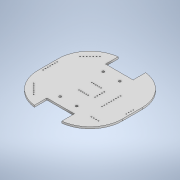
# Autodesk Inventor part: board_base
Saved by Autodesk Inventor 2020.3 (Build 243373000, 373)
## iProperties
Created: 2021-03-17
Part Number: board_base
Material: Ogólny
Document SubType Name: Modeling
Designer: patry
Density: 1 g/cm^3
Appearance: Domyślna
Author: patry
Autodesk Inventor part; units mm, degrees
ref_plane "YZ Plane" through (0, 0, 0) normal (1, 0, 0) x (0, 1, 0)
ref_plane "XZ Plane" through (0, 0, 0) normal (0, 1, 0) x (-1, 0, 0)
ref_plane "XY Plane" through (0, 0, 0) normal (0, 0, 1) x (1, 0, 0)
sketch "Szkic1" plane through (0, 0, 0) normal (0, 1, 0) x (-1, 0, 0)
  line L0 (11, 46) -> (-11, 46)
  line L1 (-46, 11) -> (-46, -11)
  line L2 (-11, -46) -> (11, -46)
  line L3 (46, -11) -> (46, 11)
  line L4 (46, 46) -> (-46, -46) construction
  line L5 (-46, 46) -> (46, -46) construction
  arc A0 (46, 44) -> (44, 46) centre (44, 44) ccw
  arc A1 (46, 11) -> (11, 46) centre (11, 11) ccw
  arc A2 (11, -46) -> (46, -11) centre (11, -11) ccw
  arc A3 (-46, -11) -> (-11, -46) centre (-11, -11) ccw
  arc A4 (-11, 46) -> (-46, 11) centre (-11, 11) ccw
  point P0 (0, 0)
  dimension "d0" = 92
  dimension "d1" = 92
  dimension "d3" = 35
  constraints: 12 end point, 10 point on circle, 10 point on line, 10 tangent, 5 centre point, 3 equal radius, 2 midpoint, 2 parallel, 1 horizontal, 1 perpendicular
  measures "d0" distance of L5.end L4.end
  measures "d1" distance of L4.end L5.start
  measures "d3" radius of A1
extrude "Wyciągnięcie proste1" add sketch "Szkic1" along normal blind 2
sketch "Szkic2" plane through (0, 2, 0) normal (0, 1, 0) x (1, 0, 0)
  line L0 (0, -49.4552) -> (0, 63.4462) construction
  line L1 (-44.5279, 0) -> (46.4745, 0) construction
  line L2 (15, 32) -> (-15, 32)
  line L3 (-15, 32) -> (-15, 46)
  line L4 (-15, 46) -> (15, 46)
  line L5 (15, 46) -> (15, 32)
  line L6 (15, 32) -> (-15, 46) construction
  line L7 (-15, 32) -> (15, 46) construction
  arc A0 (11, -46) -> (46, -11) centre (11, -11) ccw projected
  line L8 (46, -11) -> (46, 11) projected
  arc A1 (46, 11) -> (11, 46) centre (11, 11) ccw projected
  line L9 (11, 46) -> (-11, 46) projected
  arc A2 (-11, 46) -> (-46, 11) centre (-11, 11) ccw projected
  line L10 (-46, 11) -> (-46, -11) projected
  arc A3 (-46, -11) -> (-11, -46) centre (-11, -11) ccw projected
  line L11 (-11, -46) -> (11, -46) projected
  line L12 (11, 46) -> (-11, 46) projected
  line L13 (15, -46) -> (-15, -46)
  line L14 (-15, -46) -> (-15, -32)
  line L15 (-15, -32) -> (15, -32)
  line L16 (15, -32) -> (15, -46)
  line L17 (15, -46) -> (-15, -32) construction
  line L18 (-15, -46) -> (15, -32) construction
  line L19 (-11, -46) -> (11, -46) projected
  point P0 (0, 0)
  point P1 (0, 39)
  point P2 (0, -39)
  point P3 (0, -39)
  point P4 (0, 39)
  point P5 (-16, -46)
  point P6 (16, -46)
  dimension "d6" = 30
  dimension "d7" = 14
  dimension "d8" = 30
  dimension "d9" = 14
  constraints: 28 end point, 6 midpoint, 4 horizontal, 4 parallel, 2 collinear, 2 perpendicular, 2 vertical, 2 vertical alignment, 1 point on line
  measures "d6" distance of L3.end L4.end
  measures "d7" distance of L2.end L3.end
  measures "d8" distance of L15.start L15.end
  measures "d9" distance of L18.start L15.start
extrude "Wyciągnięcie proste2" cut sketch "Szkic2" against normal blind 10 contours L2 L3 A2 L4 A1 L5 | A1 L4 L5 | L3 L4 A2 | L16 L13 A0 | A0 L11 A3 L14 L15 L16 | A3 L13 L14
sketch "Szkic3" plane through (0, 2, 0) normal (0, 1, 0) x (1, 0, 0)
  line L0 (-15, -32) -> (15, -32) projected
  line L1 (-50.9262, 0) -> (55.7428, 0) construction
  point P0 (0, 0)
  point P1 (-9, -23.5)
  point P2 (9, -23.5)
  point P3 (-9, 23.5)
  point P4 (9, 23.5)
  dimension "d12" = 8.5
  dimension "d13" = 18
  dimension "d14" = 9
  constraints: 2 end point, 2 symmetric about line, 1 horizontal, 1 horizontal alignment
  measures "d12" distance from line of L0 point (-9, -23.5)
  measures "d13" distance of point (9, -23.5) point (-9, -23.5)
  measures "d14" horizontal distance of point (0, 0) point (-9, -23.5)
hole "Otwór1" at (-9, 2, 23.5) at (9, 2, 23.5) at (-9, 2, -23.5) at (9, 2, -23.5) direction (0, -1, 0) diameter 2.4 end through all clearance for "Śruba ze łbem płaskim obrobiona" size "M2" standard "ANSI Profil metryczny M"
sketch "Szkic4" plane through (0, 2, 0) normal (0, 1, 0) x (1, 0, 0)
  line L0 (-46, 11) -> (-46, -11) projected
  circle A0 centre (0, 0) radius 43.5 construction
  line L1 (-36.1473, 25.371) -> (-25.371, 36.1473) construction
  line L2 (-25.371, 36.1473) -> (-30.7591, 30.7591) construction
  line L3 (-43.5, 7.62) -> (-43.5, -7.62) construction
  line L4 (-50.7703, 0) -> (45.9031, 0) construction
  line L5 (-36.1473, -25.371) -> (-25.371, -36.1473) construction
  line L6 (-25.371, -36.1473) -> (-30.7591, -30.7591) construction
  point P0 (-43.5, 0)
  point P1 (-43.5, 2.54)
  point P2 (-43.5, -2.54)
  point P3 (-43.5, 5.08)
  point P4 (-43.5, -5.08)
  point P5 (-34.3512, 27.167)
  point P6 (-32.5552, 28.9631)
  point P7 (-27.167, 34.3512)
  point P8 (-28.9631, 32.5552)
  point P9 (-34.3512, -27.167)
  point P10 (-32.5552, -28.9631)
  point P11 (-27.167, -34.3512)
  point P12 (-28.9631, -32.5552)
  dimension "d22" = 2.54
  dimension "d23" = 2.54
  dimension "d24" = 2.54
  dimension "d25" = 2.54
  dimension "d26" = 2.54
  dimension "d27" = 2.54
  dimension "d28" = 2.5
  dimension "d36" = 15.24
  dimension "d37" = 7.62
  dimension "d38" = 135
  dimension "d39" = 5.3882
  dimension "d40" = 1.796
  dimension "d41" = 1.796
  dimension "d42" = 1.796
  dimension "d43" = 1.796
  constraints: 12 end point, 10 symmetric about line, 8 point on line, 7 coincident, 6 vertical alignment, 2 midpoint, 2 point on circle, 1 centre point, 1 horizontal, 1 horizontal alignment, 1 tangent, 1 vertical
  measures "d22" distance of A0.start point (-43.5, -2.54)
  measures "d23" distance of point (-43.5, 2.54) A0.start
  measures "d24" distance of point (-43.5, 5.08) point (-43.5, 2.54)
  measures "d25" distance of L3.start point (-43.5, 5.08)
  measures "d26" distance of point (-43.5, -5.08) point (-43.5, -2.54)
  measures "d27" distance of L3.end point (-43.5, -5.08)
  measures "d28" distance from line of L0 point (-43.5, -5.08)
  measures "d36" distance of L1.start L1.end
  measures "d37" distance of L2.start L2.end
  measures "d38" angle of L3 L1
  measures "d39" horizontal distance of L2.start L2.end
  measures "d40" horizontal distance of L2.start point (-27.167, 34.351)
  measures "d41" horizontal distance of A0.end point (-28.963, 32.555)
  measures "d42" horizontal distance of A0.end point (-32.555, 28.963)
  measures "d43" horizontal distance of point (-34.351, 27.167) point (-36.147, 25.371)
hole "Otwór2" at (-43.5, 2, 0) at (-43.5, 2, -2.54) at (-43.5, 2, 2.54) at (-43.5, 2, -5.08) at (-43.5, 2, 5.08) at (-43.5, 2, 7.62) at (-43.5, 2, -7.62) at (-36.1473, 2, 25.371) at (-30.7591, 2, 30.7591) at (-34.3512, 2, 27.167) at (-32.5552, 2, 28.9631) at (-27.167, 2, 34.3512) at (-28.9631, 2, 32.5552) at (-25.371, 2, 36.1473) at (-28.9631, 2, -32.5552) at (-27.167, 2, -34.3512) at (-32.5552, 2, -28.9631) at (-34.3512, 2, -27.167) at (-30.7591, 2, -30.7591) at (-25.371, 2, -36.1473) at (-36.1473, 2, -25.371) direction (0, -1, 0) diameter 1 end through all
sketch "Szkic5" plane through (0, 2, 0) normal (0, 1, 0) x (1, 0, 0)
  circle A0 centre (-25.371, 36.1473) radius 0.5 projected
  circle A1 centre (-34.3512, 27.167) radius 0.5 projected
  circle A2 centre (-27.167, 34.3512) radius 0.5 projected
  circle A3 centre (-25.371, -36.1473) radius 0.5 projected
  circle A4 centre (-27.167, -34.3512) radius 0.5 projected
  circle A5 centre (-34.3512, -27.167) radius 0.5 projected
  circle A6 centre (-36.1473, -25.371) radius 0.5 projected
  circle A7 centre (-43.5, -7.62) radius 0.5 projected
  circle A8 centre (-43.5, 5.08) radius 0.5 projected
  circle A9 centre (-43.5, 2.54) radius 0.5 projected
  circle A10 centre (-43.5, 0) radius 0.5 projected
  circle A11 centre (-43.5, -2.54) radius 0.5 projected
  circle A12 centre (-43.5, -5.08) radius 0.5 projected
  circle A13 centre (-43.5, 7.62) radius 0.5 projected
  circle A14 centre (-30.7591, -30.7591) radius 0.5 projected
  circle A15 centre (-32.5552, -28.9631) radius 0.5 projected
  circle A16 centre (-28.9631, -32.5552) radius 0.5 projected
  circle A17 centre (-28.9631, 32.5552) radius 0.5 projected
  circle A18 centre (-32.5552, 28.9631) radius 0.5 projected
  circle A19 centre (-30.7591, 30.7591) radius 0.5 projected
  circle A20 centre (-36.1473, 25.371) radius 0.5 projected
  circle A21 centre (-9, 23.5) radius 1.2 projected
  circle A22 centre (-9, -23.5) radius 1.2 projected
  circle A23 centre (9, -23.5) radius 1.2 projected
  circle A24 centre (9, 23.5) radius 1.2 projected
  line L0 (-15, 32) -> (-15, 45.7707) projected
  arc A25 (-15, 45.7707) -> (-46, 11) centre (-11, 11) ccw projected
  line L1 (-46, 11) -> (-46, -11) projected
  arc A26 (-46, -11) -> (-15, -45.7707) centre (-11, -11) ccw projected
  line L2 (-15, -45.7707) -> (-15, -32) projected
  line L3 (-15, -32) -> (15, -32) projected
  line L4 (15, -32) -> (15, -45.7707) projected
  arc A27 (15, -45.7707) -> (46, -11) centre (11, -11) ccw projected
  line L5 (46, -11) -> (46, 11) projected
  arc A28 (46, 11) -> (15, 45.7707) centre (11, 11) ccw projected
  line L6 (15, 45.7707) -> (15, 32) projected
  line L7 (15, 32) -> (-15, 32) projected
  line L8 (7.5, -32) -> (-7.5, -32)
  line L9 (-7.5, -32) -> (-7.5, -18.75)
  line L10 (-7.5, -18.75) -> (7.5, -18.75)
  line L11 (7.5, -18.75) -> (7.5, -32)
  line L12 (7.5, -32) -> (-7.5, -18.75) construction
  line L13 (-7.5, -32) -> (7.5, -18.75) construction
  line L14 (-15, -32) -> (15, -32) projected
  circle A29 centre (-9, -23.5) radius 4.25
  line L15 (-9, -19.25) -> (-7.5, -19.25)
  line L16 (-9, -27.75) -> (-7.5, -27.75)
  circle A30 centre (9, -23.5) radius 1.2 projected
  circle A31 centre (9, -23.5) radius 4.25
  line L17 (9, -19.25) -> (7.5, -19.25)
  line L18 (9, -27.75) -> (7.5, -27.75)
  line L19 (6, -18.75) -> (-6, -18.75)
  line L20 (-6, -18.75) -> (-6, -10.25)
  line L21 (-6, -10.25) -> (6, -10.25)
  line L22 (6, -10.25) -> (6, -18.75)
  line L23 (6, -18.75) -> (-6, -10.25) construction
  line L24 (-6, -18.75) -> (6, -10.25) construction
  line L25 (0.5, -10.25) -> (-0.5, -10.25)
  line L26 (-0.5, -10.25) -> (-0.5, -5.25)
  line L27 (-0.5, -5.25) -> (0.5, -5.25)
  line L28 (0.5, -5.25) -> (0.5, -10.25)
  line L29 (0.5, -10.25) -> (-0.5, -5.25) construction
  line L30 (-0.5, -10.25) -> (0.5, -5.25) construction
  line L31 (-48.5218, 0) -> (66.2136, 0) construction
  circle A32 centre (-9, 23.5) radius 1.2
  circle A33 centre (9, 23.5) radius 1.2
  line L32 (7.5, 32) -> (-7.5, 32)
  line L33 (-7.5, 32) -> (-7.5, 18.75)
  line L34 (-7.5, 18.75) -> (7.5, 18.75)
  line L35 (7.5, 18.75) -> (7.5, 32)
  line L36 (7.5, 32) -> (-7.5, 18.75) construction
  line L37 (-7.5, 32) -> (7.5, 18.75) construction
  line L38 (-9, 19.25) -> (-7.5, 19.25)
  line L39 (-9, 27.75) -> (-7.5, 27.75)
  circle A34 centre (9, 23.5) radius 1.2
  circle A35 centre (9, 23.5) radius 4.25
  line L40 (9, 19.25) -> (7.5, 19.25)
  line L41 (9, 27.75) -> (7.5, 27.75)
  line L42 (6, 18.75) -> (-6, 18.75)
  line L43 (-6, 18.75) -> (-6, 10.25)
  line L44 (-6, 10.25) -> (6, 10.25)
  line L45 (6, 10.25) -> (6, 18.75)
  line L46 (6, 18.75) -> (-6, 10.25) construction
  line L47 (-6, 18.75) -> (6, 10.25) construction
  line L48 (0.5, 10.25) -> (-0.5, 10.25)
  line L49 (-0.5, 10.25) -> (-0.5, 5.25)
  line L50 (-0.5, 5.25) -> (0.5, 5.25)
  line L51 (0.5, 5.25) -> (0.5, 10.25)
  line L52 (0.5, 10.25) -> (-0.5, 5.25) construction
  line L53 (-0.5, 10.25) -> (0.5, 5.25) construction
  circle A36 centre (-9, 23.5) radius 4.25
  point P0 (0, 0)
  point P1 (0, -25.375)
  point P2 (0, -25.375)
  point P3 (0, -14.5)
  point P4 (0, -14.5)
  point P5 (0, -25.375)
  point P6 (0, -7.75)
  point P7 (0, -7.75)
  point P8 (-1, -7)
  point P9 (-3, -7)
  point P10 (-5, -7)
  point P11 (1, -7)
  point P12 (3, -7)
  point P13 (5, -7)
  point P14 (0, 25.375)
  point P15 (0, 25.375)
  point P16 (0, 14.5)
  point P17 (0, 14.5)
  point P18 (0, 25.375)
  point P19 (0, 7.75)
  point P20 (0, 7.75)
  point P21 (-1, 7)
  point P22 (-3, 7)
  point P23 (-5, 7)
  point P24 (1, 7)
  point P25 (3, 7)
  point P26 (5, 7)
  dimension "d44" = 15
  dimension "d45" = 13.25
  dimension "d46" = 8.5
  dimension "d47" = 8.5
  dimension "d48" = 12
  dimension "d49" = 8.5
  dimension "d50" = 1
  dimension "d51" = 5
  dimension "d53" = 2
  dimension "d54" = 2
  dimension "d55" = 2
  dimension "d56" = 2
  dimension "d57" = 2
  dimension "d58" = 1
  dimension "d59" = 3.25
  constraints: 90 end point, 39 symmetric about line, 16 midpoint, 8 point on line, 7 centre point, 7 perpendicular, 6 parallel, 6 point on circle, 5 horizontal alignment, 4 coincident, 4 horizontal, 3 collinear, 3 vertical alignment, 5 other
  measures "d44" distance of L9.end L10.end
  measures "d45" distance of L8.end L9.end
  measures "d46" diameter of A29
  measures "d47" diameter of A31
  measures "d48" distance of L20.end L21.end
  measures "d49" distance of L19.end L20.end
  measures "d50" distance of L26.end L27.end
  measures "d51" distance of L25.end L26.end
  measures "d53" distance of point (1, -7) point (-1, -7)
  measures "d54" distance of point (-1, -7) point (-3, -7)
  measures "d55" distance of point (-3, -7) point (-5, -7)
  measures "d56" distance of point (1, -7) point (3, -7)
  measures "d57" distance of point (3, -7) point (5, -7)
  measures "d58" horizontal distance of point (-1, -7) point (0, -7.75)
  measures "d59" distance from line of L21 point (-1, -7)
hole "Otwór3" at (-1, 2, 7) at (-3, 2, 7) at (-5, 2, 7) at (1, 2, 7) at (3, 2, 7) at (5, 2, 7) at (5, 2, -7) at (3, 2, -7) at (1, 2, -7) at (-5, 2, -7) at (-3, 2, -7) at (-1, 2, -7) direction (0, -1, 0) diameter 1 end through all
sketch "Szkic6" plane through (0, 2, 0) normal (0, 1, 0) x (1, 0, 0)
  circle A0 centre (-3, 7) radius 0.5 projected
  circle A1 centre (1, 7) radius 0.5 projected
  circle A2 centre (5, 7) radius 0.5 projected
  circle A3 centre (3, -7) radius 0.5 projected
  circle A4 centre (-5, -7) radius 0.5 projected
  circle A5 centre (-1, -7) radius 0.5 projected
  circle A6 centre (-3, -7) radius 0.5 projected
  circle A7 centre (1, -7) radius 0.5 projected
  circle A8 centre (5, -7) radius 0.5 projected
  circle A9 centre (3, 7) radius 0.5 projected
  circle A10 centre (-5, 7) radius 0.5 projected
  circle A11 centre (-1, 7) radius 0.5 projected
  circle A12 centre (-25.371, 36.1473) radius 0.5 projected
  circle A13 centre (-34.3512, 27.167) radius 0.5 projected
  circle A14 centre (-27.167, 34.3512) radius 0.5 projected
  circle A15 centre (-25.371, -36.1473) radius 0.5 projected
  circle A16 centre (-27.167, -34.3512) radius 0.5 projected
  circle A17 centre (-34.3512, -27.167) radius 0.5 projected
  circle A18 centre (-36.1473, -25.371) radius 0.5 projected
  circle A19 centre (-43.5, -7.62) radius 0.5 projected
  circle A20 centre (-43.5, 5.08) radius 0.5 projected
  circle A21 centre (-43.5, 2.54) radius 0.5 projected
  circle A22 centre (-43.5, 0) radius 0.5 projected
  circle A23 centre (-43.5, -2.54) radius 0.5 projected
  circle A24 centre (-43.5, -5.08) radius 0.5 projected
  circle A25 centre (-43.5, 7.62) radius 0.5 projected
  circle A26 centre (-30.7591, -30.7591) radius 0.5 projected
  circle A27 centre (-32.5552, -28.9631) radius 0.5 projected
  circle A28 centre (-28.9631, -32.5552) radius 0.5 projected
  circle A29 centre (-28.9631, 32.5552) radius 0.5 projected
  circle A30 centre (-32.5552, 28.9631) radius 0.5 projected
  circle A31 centre (-30.7591, 30.7591) radius 0.5 projected
  circle A32 centre (-36.1473, 25.371) radius 0.5 projected
  circle A33 centre (-9, 23.5) radius 1.2 projected
  circle A34 centre (-9, -23.5) radius 1.2 projected
  circle A35 centre (9, -23.5) radius 1.2 projected
  circle A36 centre (9, 23.5) radius 1.2 projected
  line L0 (-15, 32) -> (-15, 45.7707) projected
  arc A37 (-15, 45.7707) -> (-46, 11) centre (-11, 11) ccw projected
  line L1 (-46, 11) -> (-46, -11) projected
  arc A38 (-46, -11) -> (-15, -45.7707) centre (-11, -11) ccw projected
  line L2 (-15, -45.7707) -> (-15, -32) projected
  line L3 (-15, -32) -> (15, -32) projected
  line L4 (15, -32) -> (15, -45.7707) projected
  arc A39 (15, -45.7707) -> (46, -11) centre (11, -11) ccw projected
  line L5 (46, -11) -> (46, 11) projected
  arc A40 (46, 11) -> (15, 45.7707) centre (11, 11) ccw projected
  line L6 (15, 45.7707) -> (15, 32) projected
  line L7 (15, 32) -> (-15, 32) projected
  line L8 (25.8, -12.7) -> (8, -12.7)
  line L9 (8, -12.7) -> (8, 12.7)
  line L10 (8, 12.7) -> (25.8, 12.7)
  line L11 (25.8, 12.7) -> (25.8, -12.7)
  line L12 (25.8, -12.7) -> (8, 12.7) construction
  line L13 (8, -12.7) -> (25.8, 12.7) construction
  line L14 (6, 10.25) -> (6, 18.75) projected
  line L15 (6, -10.25) -> (6, -18.75) projected
  point P0 (0, 0)
  point P1 (16.9, 0)
  point P2 (16.9, 0)
  point P3 (10.55, 0)
  point P4 (23.25, 0)
  point P5 (10.55, 2.54)
  point P6 (10.55, 5.08)
  point P7 (10.55, -2.54)
  point P8 (10.55, -5.08)
  point P9 (23.25, 0)
  point P10 (23.25, 2.54)
  point P11 (23.25, 5.08)
  point P12 (23.25, -2.54)
  point P13 (23.25, -5.08)
  point P14 (23.25, 7.62)
  point P15 (23.25, 10.16)
  point P16 (23.25, -7.62)
  point P17 (23.25, -10.16)
  dimension "d67" = 17.8
  dimension "d68" = 25.4
  dimension "d69" = 2
  dimension "d70" = 6.35
  dimension "d71" = 6.35
  dimension "d72" = 2.54
  dimension "d73" = 2.54
  dimension "d74" = 2.54
  dimension "d75" = 2.54
  dimension "d76" = 2.54
  dimension "d77" = 2.54
  dimension "d78" = 2.54
  dimension "d79" = 2.54
  dimension "d80" = 2.54
  dimension "d82" = 2.54
  dimension "d83" = 2.54
  dimension "d85" = 2.54
  constraints: 12 end point, 12 vertical alignment, 3 midpoint, 2 parallel, 1 coincident, 1 horizontal, 1 horizontal alignment, 1 perpendicular
  measures "d67" distance of L9.end L10.end
  measures "d68" distance of L8.end L9.end
  measures "d69" distance between parallel lines of L9 L14
  measures "d70" distance of point (16.9, 0) point (10.55, 0)
  measures "d71" distance of point (16.9, 0) point (23.25, 0)
  measures "d72" distance of point (10.55, 2.54) point (10.55, 0)
  measures "d73" distance of point (10.55, 2.54) point (10.55, 5.08)
  measures "d74" distance of point (10.55, 0) point (10.55, -2.54)
  measures "d75" distance of point (10.55, -2.54) point (10.55, -5.08)
  measures "d76" distance of point (23.25, 2.54) point (23.25, 0)
  measures "d77" distance of point (23.25, 2.54) point (23.25, 5.08)
  measures "d78" distance of point (23.25, 0) point (23.25, -2.54)
  measures "d79" distance of point (23.25, -2.54) point (23.25, -5.08)
  measures "d80" distance of point (23.25, 10.16) point (23.25, 7.62)
  measures "d82" distance of point (23.25, 5.08) point (23.25, 7.62)
  measures "d83" distance of point (23.25, -10.16) point (23.25, -7.62)
  measures "d85" distance of point (23.25, -5.08) point (23.25, -7.62)
hole "Otwór4" at (10.55, 2, 5.08) at (10.55, 2, 2.54) at (10.55, 2, -5.08) at (10.55, 2, -2.54) at (10.55, 2, 0) at (23.25, 2, 7.62) at (23.25, 2, 10.16) at (23.25, 2, -7.62) at (23.25, 2, -10.16) at (23.25, 2, 0) at (23.25, 2, -2.54) at (23.25, 2, -5.08) at (23.25, 2, 2.54) at (23.25, 2, 5.08) direction (0, -1, 0) diameter 1 end through all
sketch "Szkic7" plane through (0, 2, 0) normal (0, 1, 0) x (1, 0, 0)
  circle A0 centre (23.25, -2.54) radius 0.5 projected
  circle A1 centre (23.25, 2.54) radius 0.5 projected
  circle A2 centre (23.25, 10.16) radius 0.5 projected
  circle A3 centre (23.25, -10.16) radius 0.5 projected
  circle A4 centre (10.55, 0) radius 0.5 projected
  circle A5 centre (10.55, 5.08) radius 0.5 projected
  circle A6 centre (10.55, -5.08) radius 0.5 projected
  circle A7 centre (10.55, -2.54) radius 0.5 projected
  circle A8 centre (10.55, 2.54) radius 0.5 projected
  circle A9 centre (23.25, -7.62) radius 0.5 projected
  circle A10 centre (23.25, 7.62) radius 0.5 projected
  circle A11 centre (23.25, 0) radius 0.5 projected
  circle A12 centre (23.25, 5.08) radius 0.5 projected
  circle A13 centre (23.25, -5.08) radius 0.5 projected
  circle A14 centre (-3, 7) radius 0.5 projected
  circle A15 centre (1, 7) radius 0.5 projected
  circle A16 centre (5, 7) radius 0.5 projected
  circle A17 centre (3, -7) radius 0.5 projected
  circle A18 centre (-5, -7) radius 0.5 projected
  circle A19 centre (-1, -7) radius 0.5 projected
  circle A20 centre (-3, -7) radius 0.5 projected
  circle A21 centre (1, -7) radius 0.5 projected
  circle A22 centre (5, -7) radius 0.5 projected
  circle A23 centre (3, 7) radius 0.5 projected
  circle A24 centre (-5, 7) radius 0.5 projected
  circle A25 centre (-1, 7) radius 0.5 projected
  circle A26 centre (-25.371, 36.1473) radius 0.5 projected
  circle A27 centre (-34.3512, 27.167) radius 0.5 projected
  circle A28 centre (-27.167, 34.3512) radius 0.5 projected
  circle A29 centre (-25.371, -36.1473) radius 0.5 projected
  circle A30 centre (-27.167, -34.3512) radius 0.5 projected
  circle A31 centre (-34.3512, -27.167) radius 0.5 projected
  circle A32 centre (-36.1473, -25.371) radius 0.5 projected
  circle A33 centre (-43.5, -7.62) radius 0.5 projected
  circle A34 centre (-43.5, 5.08) radius 0.5 projected
  circle A35 centre (-43.5, 2.54) radius 0.5 projected
  circle A36 centre (-43.5, 0) radius 0.5 projected
  circle A37 centre (-43.5, -2.54) radius 0.5 projected
  circle A38 centre (-43.5, -5.08) radius 0.5 projected
  circle A39 centre (-43.5, 7.62) radius 0.5 projected
  circle A40 centre (-30.7591, -30.7591) radius 0.5 projected
  circle A41 centre (-32.5552, -28.9631) radius 0.5 projected
  circle A42 centre (-28.9631, -32.5552) radius 0.5 projected
  circle A43 centre (-28.9631, 32.5552) radius 0.5 projected
  circle A44 centre (-32.5552, 28.9631) radius 0.5 projected
  circle A45 centre (-30.7591, 30.7591) radius 0.5 projected
  circle A46 centre (-36.1473, 25.371) radius 0.5 projected
  circle A47 centre (-9, 23.5) radius 1.2 projected
  circle A48 centre (-9, -23.5) radius 1.2 projected
  circle A49 centre (9, -23.5) radius 1.2 projected
  circle A50 centre (9, 23.5) radius 1.2 projected
  line L0 (-15, 32) -> (-15, 45.7707) projected
  arc A51 (-15, 45.7707) -> (-46, 11) centre (-11, 11) ccw projected
  line L1 (-46, 11) -> (-46, -11) projected
  arc A52 (-46, -11) -> (-15, -45.7707) centre (-11, -11) ccw projected
  line L2 (-15, -45.7707) -> (-15, -32) projected
  line L3 (-15, -32) -> (15, -32) projected
  line L4 (15, -32) -> (15, -45.7707) projected
  arc A53 (15, -45.7707) -> (46, -11) centre (11, -11) ccw projected
  line L5 (46, -11) -> (46, 11) projected
  arc A54 (46, 11) -> (15, 45.7707) centre (11, 11) ccw projected
  line L6 (15, 45.7707) -> (15, 32) projected
  line L7 (15, 32) -> (-15, 32) projected
  line L8 (-48.5218, 0) -> (66.2136, 0) construction
  point P0 (0, 0)
  point P1 (43.5, -1.27)
  point P2 (43.5, 1.27)
  point P3 (43.5, 3.81)
  point P4 (43.5, -3.81)
  dimension "d93" = 2.5
  dimension "d94" = 2.54
  dimension "d95" = 1.27
  dimension "d96" = 2.54
  dimension "d97" = 2.54
  constraints: 3 vertical alignment
  measures "d93" distance from line of L5 point (43.5, -1.27)
  measures "d94" distance of point (43.5, 1.27) point (43.5, -1.27)
  measures "d95" distance from line of L8 point (43.5, 1.27)
  measures "d96" distance of point (43.5, 3.81) point (43.5, 1.27)
  measures "d97" distance of point (43.5, -3.81) point (43.5, -1.27)
hole "Otwór5" at (43.5, 2, 3.81) at (43.5, 2, -3.81) at (43.5, 2, -1.27) at (43.5, 2, 1.27) direction (0, -1, 0) diameter 1 end through all
sketch "Szkic8" plane through (0, 2, 0) normal (0, 1, 0) x (1, 0, 0)
  line L0 (27.0445, -22.5) -> (42.0445, -22.5) construction
  line L1 (42.0445, -22.5) -> (42.0445, 22.5) construction
  line L2 (42.0445, 22.5) -> (27.0445, 22.5) construction
  line L3 (27.0445, 22.5) -> (27.0445, -22.5) construction
  line L4 (27.0445, -22.5) -> (42.0445, 22.5) construction
  line L5 (42.0445, -22.5) -> (27.0445, 22.5) construction
  point P0 (0, 0)
  point P1 (34.5445, 0)
  point P2 (27.0445, -25.5)
  point P3 (29.5845, -25.5)
  point P4 (32.1245, -25.5)
  point P5 (34.6645, -25.5)
  dimension "d105" = 15
  dimension "d106" = 45
  dimension "d107" = 2.54
  dimension "d108" = 2.54
  dimension "d109" = 2.54
  dimension "d110" = 3
  dimension "d111" = 0
  constraints: 12 end point, 3 horizontal alignment, 2 midpoint, 2 parallel, 1 horizontal, 1 perpendicular
  measures "d105" distance of L2.end L1.end
  measures "d106" distance of L1.end L0.end
  measures "d107" distance of point (29.585, -25.5) point (27.045, -25.5)
  measures "d108" distance of point (32.125, -25.5) point (29.585, -25.5)
  measures "d109" distance of point (34.665, -25.5) point (32.125, -25.5)
  measures "d110" distance from line of L0 point (27.045, -25.5)
  measures "d111" distance from line of L3 point (27.045, -25.5)
hole "Otwór6" at (34.6645, 2, 25.5) at (32.1245, 2, 25.5) at (29.5845, 2, 25.5) at (27.0445, 2, 25.5) direction (0, -1, 0) diameter 1 end through all
sketch "Szkic9" plane through (0, 2, 0) normal (0, 1, 0) x (1, 0, 0)
  circle A0 centre (29.5845, -25.5) radius 0.5 projected
  circle A1 centre (34.6645, -25.5) radius 0.5 projected
  circle A2 centre (32.1245, -25.5) radius 0.5 projected
  circle A3 centre (27.0445, -25.5) radius 0.5 projected
  circle A4 centre (43.5, 1.27) radius 0.5 projected
  circle A5 centre (43.5, -3.81) radius 0.5 projected
  circle A6 centre (43.5, 3.81) radius 0.5 projected
  circle A7 centre (43.5, -1.27) radius 0.5 projected
  circle A8 centre (23.25, -2.54) radius 0.5 projected
  circle A9 centre (23.25, 2.54) radius 0.5 projected
  circle A10 centre (23.25, 10.16) radius 0.5 projected
  circle A11 centre (23.25, -10.16) radius 0.5 projected
  circle A12 centre (10.55, 0) radius 0.5 projected
  circle A13 centre (10.55, 5.08) radius 0.5 projected
  circle A14 centre (10.55, -5.08) radius 0.5 projected
  circle A15 centre (10.55, -2.54) radius 0.5 projected
  circle A16 centre (10.55, 2.54) radius 0.5 projected
  circle A17 centre (23.25, -7.62) radius 0.5 projected
  circle A18 centre (23.25, 7.62) radius 0.5 projected
  circle A19 centre (23.25, 0) radius 0.5 projected
  circle A20 centre (23.25, 5.08) radius 0.5 projected
  circle A21 centre (23.25, -5.08) radius 0.5 projected
  circle A22 centre (-3, 7) radius 0.5 projected
  circle A23 centre (1, 7) radius 0.5 projected
  circle A24 centre (5, 7) radius 0.5 projected
  circle A25 centre (3, -7) radius 0.5 projected
  circle A26 centre (-5, -7) radius 0.5 projected
  circle A27 centre (-1, -7) radius 0.5 projected
  circle A28 centre (-3, -7) radius 0.5 projected
  circle A29 centre (1, -7) radius 0.5 projected
  circle A30 centre (5, -7) radius 0.5 projected
  circle A31 centre (3, 7) radius 0.5 projected
  circle A32 centre (-5, 7) radius 0.5 projected
  circle A33 centre (-1, 7) radius 0.5 projected
  circle A34 centre (-25.371, 36.1473) radius 0.5 projected
  circle A35 centre (-34.3512, 27.167) radius 0.5 projected
  circle A36 centre (-27.167, 34.3512) radius 0.5 projected
  circle A37 centre (-25.371, -36.1473) radius 0.5 projected
  circle A38 centre (-27.167, -34.3512) radius 0.5 projected
  circle A39 centre (-34.3512, -27.167) radius 0.5 projected
  circle A40 centre (-36.1473, -25.371) radius 0.5 projected
  circle A41 centre (-43.5, -7.62) radius 0.5 projected
  circle A42 centre (-43.5, 5.08) radius 0.5 projected
  circle A43 centre (-43.5, 2.54) radius 0.5 projected
  circle A44 centre (-43.5, 0) radius 0.5 projected
  circle A45 centre (-43.5, -2.54) radius 0.5 projected
  circle A46 centre (-43.5, -5.08) radius 0.5 projected
  circle A47 centre (-43.5, 7.62) radius 0.5 projected
  circle A48 centre (-30.7591, -30.7591) radius 0.5 projected
  circle A49 centre (-32.5552, -28.9631) radius 0.5 projected
  circle A50 centre (-28.9631, -32.5552) radius 0.5 projected
  circle A51 centre (-28.9631, 32.5552) radius 0.5 projected
  circle A52 centre (-32.5552, 28.9631) radius 0.5 projected
  circle A53 centre (-30.7591, 30.7591) radius 0.5 projected
  circle A54 centre (-36.1473, 25.371) radius 0.5 projected
  circle A55 centre (-9, 23.5) radius 1.2 projected
  circle A56 centre (-9, -23.5) radius 1.2 projected
  circle A57 centre (9, -23.5) radius 1.2 projected
  circle A58 centre (9, 23.5) radius 1.2 projected
  line L0 (-15, 32) -> (-15, 45.7707) projected
  arc A59 (-15, 45.7707) -> (-46, 11) centre (-11, 11) ccw projected
  line L1 (-46, 11) -> (-46, -11) projected
  arc A60 (-46, -11) -> (-15, -45.7707) centre (-11, -11) ccw projected
  line L2 (-15, -45.7707) -> (-15, -32) projected
  line L3 (-15, -32) -> (15, -32) projected
  line L4 (15, -32) -> (15, -45.7707) projected
  arc A61 (15, -45.7707) -> (46, -11) centre (11, -11) ccw projected
  line L5 (46, -11) -> (46, 11) projected
  arc A62 (46, 11) -> (15, 45.7707) centre (11, 11) ccw projected
  line L6 (15, 45.7707) -> (15, 32) projected
  line L7 (15, 32) -> (-15, 32) projected
  circle A63 centre (-9, 23.5) radius 4.25 projected
  circle A64 centre (9, 23.5) radius 4.25 projected
  line L8 (7.5, 18.75) -> (7.5, 32) projected
  line L9 (-7.5, 32) -> (-7.5, 18.75) projected
  line L10 (6, 18.75) -> (-6, 18.75) projected
  line L11 (-6, 18.75) -> (-6, 10.25) projected
  line L12 (-6, 10.25) -> (6, 10.25) projected
  line L13 (6, 10.25) -> (6, 18.75) projected
  circle A65 centre (-9, -23.5) radius 4.25 projected
  circle A66 centre (9, -23.5) radius 4.25 projected
  line L14 (7.5, -18.75) -> (7.5, -32) projected
  line L15 (-7.5, -32) -> (-7.5, -18.75) projected
  line L16 (-6, -18.75) -> (-6, -10.25) projected
  line L17 (-7.5, -18.75) -> (7.5, -18.75) projected
  line L18 (6, -10.25) -> (6, -18.75) projected
  line L19 (-6, -10.25) -> (6, -10.25) projected
  line L20 (0.5, 5.25) -> (0.5, 10.25) projected
  line L21 (-0.5, 10.25) -> (-0.5, 5.25) projected
  line L22 (-0.5, 5.25) -> (0.5, 5.25) projected
  line L23 (-0.5, -5.25) -> (0.5, -5.25) projected
  line L24 (-0.5, -10.25) -> (-0.5, -5.25) projected
  line L25 (0.5, -5.25) -> (0.5, -10.25) projected
  line L26 (27.0445, 22.5) -> (27.0445, -22.5) construction
  line L27 (42.0445, 22.5) -> (27.0445, 22.5) construction
  line L28 (42.0445, -22.5) -> (42.0445, 22.5) construction
  line L29 (27.0445, -22.5) -> (42.0445, -22.5) construction
  line L30 (25.8, 12.7) -> (25.8, -12.7) projected
  line L31 (8, 12.7) -> (25.8, 12.7) projected
  line L32 (8, -12.7) -> (8, 12.7) projected
  line L33 (25.8, -12.7) -> (8, -12.7) projected
  point P0 (0, 0)
sketch "Szkic10" plane through (0, 2, 0) normal (0, 1, 0) x (1, 0, 0)
  circle A0 centre (29.5845, -25.5) radius 0.5 projected
  circle A1 centre (34.6645, -25.5) radius 0.5 projected
  circle A2 centre (32.1245, -25.5) radius 0.5 projected
  circle A3 centre (27.0445, -25.5) radius 0.5 projected
  circle A4 centre (43.5, 1.27) radius 0.5 projected
  circle A5 centre (43.5, -3.81) radius 0.5 projected
  circle A6 centre (43.5, 3.81) radius 0.5 projected
  circle A7 centre (43.5, -1.27) radius 0.5 projected
  circle A8 centre (23.25, -2.54) radius 0.5 projected
  circle A9 centre (23.25, 2.54) radius 0.5 projected
  circle A10 centre (23.25, 10.16) radius 0.5 projected
  circle A11 centre (23.25, -10.16) radius 0.5 projected
  circle A12 centre (10.55, 0) radius 0.5 projected
  circle A13 centre (10.55, 5.08) radius 0.5 projected
  circle A14 centre (10.55, -5.08) radius 0.5 projected
  circle A15 centre (10.55, -2.54) radius 0.5 projected
  circle A16 centre (10.55, 2.54) radius 0.5 projected
  circle A17 centre (23.25, -7.62) radius 0.5 projected
  circle A18 centre (23.25, 7.62) radius 0.5 projected
  circle A19 centre (23.25, 0) radius 0.5 projected
  circle A20 centre (23.25, 5.08) radius 0.5 projected
  circle A21 centre (23.25, -5.08) radius 0.5 projected
  circle A22 centre (-3, 7) radius 0.5 projected
  circle A23 centre (1, 7) radius 0.5 projected
  circle A24 centre (5, 7) radius 0.5 projected
  circle A25 centre (3, -7) radius 0.5 projected
  circle A26 centre (-5, -7) radius 0.5 projected
  circle A27 centre (-1, -7) radius 0.5 projected
  circle A28 centre (-3, -7) radius 0.5 projected
  circle A29 centre (1, -7) radius 0.5 projected
  circle A30 centre (5, -7) radius 0.5 projected
  circle A31 centre (3, 7) radius 0.5 projected
  circle A32 centre (-5, 7) radius 0.5 projected
  circle A33 centre (-1, 7) radius 0.5 projected
  circle A34 centre (-25.371, 36.1473) radius 0.5 projected
  circle A35 centre (-34.3512, 27.167) radius 0.5 projected
  circle A36 centre (-27.167, 34.3512) radius 0.5 projected
  circle A37 centre (-25.371, -36.1473) radius 0.5 projected
  circle A38 centre (-27.167, -34.3512) radius 0.5 projected
  circle A39 centre (-34.3512, -27.167) radius 0.5 projected
  circle A40 centre (-36.1473, -25.371) radius 0.5 projected
  circle A41 centre (-43.5, -7.62) radius 0.5 projected
  circle A42 centre (-43.5, 5.08) radius 0.5 projected
  circle A43 centre (-43.5, 2.54) radius 0.5 projected
  circle A44 centre (-43.5, 0) radius 0.5 projected
  circle A45 centre (-43.5, -2.54) radius 0.5 projected
  circle A46 centre (-43.5, -5.08) radius 0.5 projected
  circle A47 centre (-43.5, 7.62) radius 0.5 projected
  circle A48 centre (-30.7591, -30.7591) radius 0.5 projected
  circle A49 centre (-32.5552, -28.9631) radius 0.5 projected
  circle A50 centre (-28.9631, -32.5552) radius 0.5 projected
  circle A51 centre (-28.9631, 32.5552) radius 0.5 projected
  circle A52 centre (-32.5552, 28.9631) radius 0.5 projected
  circle A53 centre (-30.7591, 30.7591) radius 0.5 projected
  circle A54 centre (-36.1473, 25.371) radius 0.5 projected
  circle A55 centre (-9, 23.5) radius 1.2 projected
  circle A56 centre (-9, -23.5) radius 1.2 projected
  circle A57 centre (9, -23.5) radius 1.2 projected
  circle A58 centre (9, 23.5) radius 1.2 projected
  line L0 (-15, 32) -> (-15, 45.7707) projected
  arc A59 (-15, 45.7707) -> (-46, 11) centre (-11, 11) ccw projected
  line L1 (-46, 11) -> (-46, -11) projected
  arc A60 (-46, -11) -> (-15, -45.7707) centre (-11, -11) ccw projected
  line L2 (-15, -45.7707) -> (-15, -32) projected
  line L3 (-15, -32) -> (15, -32) projected
  line L4 (15, -32) -> (15, -45.7707) projected
  arc A61 (15, -45.7707) -> (46, -11) centre (11, -11) ccw projected
  line L5 (46, -11) -> (46, 11) projected
  arc A62 (46, 11) -> (15, 45.7707) centre (11, 11) ccw projected
  line L6 (15, 45.7707) -> (15, 32) projected
  line L7 (15, 32) -> (-15, 32) projected
  point P0 (0, 0)
equation "\"d0\" = d1"
equation "\"d7\" = d9"
equation "\"d23\" = d22"
equation "\"d24\" = d22"
equation "\"d25\" = d22"
equation "\"d26\" = d22"
equation "\"d27\" = d22"
equation "\"d40\" = 0.333333 * d39"
equation "\"d41\" = d40"
equation "\"d42\" = d40"
equation "\"d43\" = d41"
equation "\"d54\" = d53"
equation "\"d55\" = d54"
equation "\"d56\" = d53"
equation "\"d57\" = d56"
equation "\"d58\" = 0.5 * d54"
equation "\"d71\" = d70"
equation "\"d73\" = d72"
equation "\"d74\" = d72"
equation "\"d75\" = d74"
equation "\"d77\" = d76"
equation "\"d78\" = d76"
equation "\"d79\" = d78"
equation "\"d80\" = d81"
equation "\"d82\" = d77"
equation "\"d83\" = d84"
equation "\"d85\" = d79"
equation "\"d95\" = 0.5 * d94"
equation "\"d96\" = d94"
equation "\"d97\" = d94"
equation "\"d108\" = d107"
equation "\"d109\" = d108"
equation "\"d81\" = 2.54"
equation "\"d84\" = 2.54"
